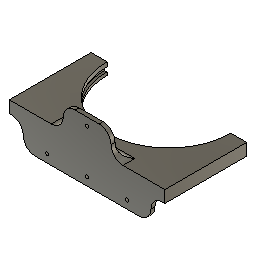
klik en klaar muurbeugel achterkant (Autodesk Fusion 360 design; units mm, degrees)
Autodesk Fusion 360 part; units mm, degrees
sketch "Sketch1" plane through (0, 0, 0) normal (0, 0, 1) x (1, 0, 0)
  circle A0 centre (0, 0) radius 87.5
  circle A1 centre (0, 0) radius 77.5
  line L0 (77.5, 0) -> (97.5, 0)
  line L1 (97.5, 0) -> (97.5, -97.5)
  line L2 (97.5, -97.5) -> (77.5, -97.5)
  line L3 (77.5, -97.5) -> (77.5, 0)
  line L4 (-77.5, 0) -> (-97.5, 0)
  line L5 (-97.5, 0) -> (-97.5, -97.5)
  line L6 (-97.5, -97.5) -> (-77.5, -97.5)
  line L7 (-77.5, -97.5) -> (-77.5, 0)
  line L8 (97.5, -97.5) -> (-97.5, -97.5)
  line L9 (-97.5, -97.5) -> (-97.5, -102.5)
  line L10 (-97.5, -102.5) -> (97.5, -102.5)
  line L11 (97.5, -102.5) -> (97.5, -97.5)
  dimension "d1" = 155
  dimension "d2" = 175
  dimension "d15" = 97.5
  dimension "d16" = 5
  dimension "d17" = 10
  dimension "d18" = 20
  dimension "d19" = 20
  constraint coincident A0.centre A1.centre
  constraint horizontal L0
  constraint vertical L1
  constraint horizontal L2
  constraint vertical L3
  constraint coincident A1 L0.start
  constraint horizontal L4
  constraint vertical L5
  constraint horizontal L6
  constraint vertical L7
  constraint coincident A1 L4.start
  constraint collinear L2 L6
  constraint horizontal L8
  constraint vertical L9
  constraint horizontal L10
  constraint vertical L11
  constraint collinear L2 L8
  constraint collinear L5 L9
  constraint collinear L1 L11
  measures "d1" diameter of A1
  measures "d2" diameter of A0
  measures "d15" distance of A0.centre L8
  measures "d16" distance of L8 L10
  measures "d17" distance of A0 A1
  measures "d18" distance of L1 L3
  measures "d19" distance of L5 L7
extrude "Extrude1" add sketch "Sketch1" along normal blind 15 contours A0 L0 L1 L2 L3 L8 | A0 L0 L3 | A0 L4 L7 | A0 L4 L5 L6 L7 L8 | A0 L3 L7 L8 | A0 A1 L3 L7 | L2 L6 L8 L9 L10 L11
sketch "Sketch2" plane through (0, 0, 0) normal (0, 0, 1) x (1, 0, 0)
  circle A0 centre (0, 0) radius 80.5
  dimension "d10" = 161
  constraint coincident A0.centre origin
  measures "d10" diameter of A0
extrude "Extrude2" cut sketch "Sketch2" along normal blind 5.5 from surface at 4
sketch "Sketch3" plane through (0, 0, 15) normal (0, 0, 1) x (-1, 0, 0)
  line L0 (77.5, 0) -> (97.5, 0)
  line L1 (97.5, 0) -> (97.5, 102.5)
  line L2 (97.5, 102.5) -> (-97.5, 102.5)
  line L3 (-97.5, 102.5) -> (-97.5, 0)
  line L4 (-97.5, 0) -> (-77.5, 0)
  arc A0 (77.5, 0) -> (-77.5, 0) centre (0, 0) ccw
  line L5 (-30, 102.5) -> (30, 102.5)
  line L6 (30, 102.5) -> (30, 97.5)
  line L7 (30, 97.5) -> (-30, 97.5)
  line L8 (-30, 97.5) -> (-30, 102.5)
  dimension "d22" = 30
  dimension "d23" = 30
  constraint horizontal L5
  constraint vertical L6
  constraint horizontal L7
  constraint vertical L8
  constraint coincident L2 L5.start
  measures "d22" distance of A0.centre L8
  measures "d23" distance of A0.centre L6
extrude "Extrude3" add sketch "Sketch3" along normal blind 30 contours L2 L5 L6 L7 L8
fillet "Fillet2" radius 15 4 edges at (-30, -100, 45) (30, -100, 45) (-30, -100, 15) (30, -100, 15)
sketch "Sketch4" plane through (0, -97.5, 0) normal (0, 1, 0) x (-1, 0, 0)
  arc A0 (-15, 45) -> (-30, 30) centre (-15, 30) ccw
  arc A1 (-45, 15) -> (-30, 30) centre (-45, 30) ccw
  line L0 (-45, 15) -> (45, 15)
  arc A2 (30, 30) -> (45, 15) centre (45, 30) ccw
  arc A3 (30, 30) -> (15, 45) centre (15, 30) ccw
  line L1 (15, 45) -> (-15, 45)
  line L2 (-97.5, 7.5) -> (97.5, 7.5) construction
  line L3 (-45, 0) -> (45, 0)
  line L4 (15, -30) -> (-15, -30)
  arc A4 (15, -30) -> (30, -15) centre (15, -15) ccw
  arc A5 (45, 0) -> (30, -15) centre (45, -15) ccw
  arc A6 (-30, -15) -> (-15, -30) centre (-15, -15) ccw
  arc A7 (-30, -15) -> (-45, 0) centre (-45, -15) ccw
  point P0 (0, 30)
  point P1 (-97.5, 7.5)
  point P2 (97.5, 7.5)
  point P3 (0, -15)
  dimension "d28" = 15
  constraint coincident P1 L2.start
  constraint coincident P2 L2.end
  constraint symmetric A0.start L2 L4.end
  constraint symmetric A0.end L2 A6.start
  constraint symmetric A0 L2 A6
  constraint symmetric A1.start L2 L3.start
  constraint symmetric A1 L2 A7
  constraint symmetric L0.end L2 L3.end
  constraint symmetric A2.start L2 A4.end
  constraint symmetric A2 L2 A5
  constraint symmetric A3.end L2 L4.start
  constraint symmetric A3 L2 A4
  constraint symmetric P0 L2 P3
  measures "d28" distance of L0 P0
sketch "Sketch5" plane through (0, 0, 0) normal (0, 0, -1) x (1, 0, 0)
  line L0 (-97.5, 0) -> (-77.5, 0)
  arc A0 (77.5, 0) -> (-77.5, 0) centre (0, 0) ccw
  line L1 (77.5, 0) -> (97.5, 0)
  line L2 (97.5, 0) -> (97.5, 102.5)
  line L3 (97.5, 102.5) -> (-97.5, 102.5)
  line L4 (-97.5, 102.5) -> (-97.5, 0)
  line L5 (80, 102.5) -> (-80, 102.5)
  line L6 (-80, 102.5) -> (-80, 97.5)
  line L7 (-80, 97.5) -> (80, 97.5)
  line L8 (80, 97.5) -> (80, 102.5)
  dimension "d39" = 80
  dimension "d40" = 80
  constraint horizontal L5
  constraint vertical L6
  constraint horizontal L7
  constraint vertical L8
  constraint coincident L3 L5.start
  measures "d39" distance of A0.centre L8
  measures "d40" distance of A0.centre L6
extrude "Extrude4" add sketch "Sketch5" along normal blind 30 contours L3 L5 L6 L7 L8
fillet "Fillet4" radius 15 4 edges at (80, -100, -30) (-80, -100, -30) (-80, -100, 0) (80, -100, 0)
sketch "Sketch6" plane through (0, -97.5, 0) normal (0, 1, 0) x (-1, 0, 0)
  arc A0 (65, -30) -> (80, -15) centre (65, -15) ccw
  arc A1 (95, 0) -> (80, -15) centre (95, -15) ccw
  line L0 (95, 0) -> (-95, 0)
  arc A2 (-80, -15) -> (-95, 0) centre (-95, -15) ccw
  arc A3 (-80, -15) -> (-65, -30) centre (-65, -15) ccw
  line L1 (-65, -30) -> (65, -30)
  line L2 (-77.5, 15) -> (77.5, 15)
  point P0 (0, -20)
  point P1 (0, 35)
  point P2 (50, -20)
  point P3 (-50, -20)
  dimension "d49" = 20
  dimension "d50" = 20
  dimension "d53" = 50
  dimension "d54" = 50
  measures "d49" distance of L0 P0
  measures "d50" distance of P1 L2
  measures "d53" distance of P0 P3
  measures "d54" distance of P0 P2
hole "Hole2" at (0, -97.5, -20) at (0, -97.5, 35) at (-50, -97.5, -20) at (50, -97.5, -20) direction (0, -1, 0) diameter 4 end through all countersink diameter 4.4 countersink angle 90
sketch "Sketch7" plane through (0, 0, 0) normal (0, 1, 0) x (-1, 0, 0)
  line L0 (77.5, 9.5) -> (80.5, 9.5)
  line L1 (80.5, 9.5) -> (80.5, 4)
  line L2 (80.5, 4) -> (77.5, 4)
  line L3 (77.5, 4) -> (77.5, 0)
  line L4 (77.5, 0) -> (97.5, 0)
  line L5 (97.5, 0) -> (97.5, 15)
  line L6 (97.5, 15) -> (77.5, 15)
  line L7 (77.5, 15) -> (77.5, 9.5)
  line L8 (-77.5, 0) -> (-97.5, 0)
  line L9 (-97.5, 0) -> (-97.5, 15)
  point P0 (90, 7.5)
  point P1 (-90, 7.5)
  dimension "d55" = 7.5
  dimension "d56" = 7.5
  dimension "d57" = 7.5
  dimension "d58" = 7.5
  measures "d55" distance of P1 L8
  measures "d56" distance of L4 P0
  measures "d57" distance of L5 P0
  measures "d58" distance of P1 L9
hole "Hole3" at (-90, 0, 7.5) at (90, 0, 7.5) direction (0, -1, 0) diameter 3.5 depth 50 tip angle 180
fillet "Fillet5" radius 10 2 edges at (0, -97.5, 0) (0, -97.5, 15)
equation "d15 = d2 / 2 + 10 mm"
equation "d18 = d17 + 10 mm"
equation "d19 = d18"
equation "d23 = d22"
equation "d40 = d39"
equation "d56 = d55"
equation "d58 = d57"
